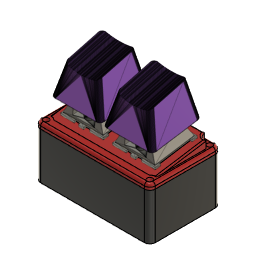
BFDeck x2 v6 (Autodesk Fusion 360 design; units mm, degrees)
Autodesk Fusion 360 part; units mm, degrees
sketch "Sketch1" plane through (0, 0, 0) normal (0, 0, 1) x (1, 0, 0)
  line L0 (2, 0) -> (40, 0)
  line L1 (42, 2) -> (42, 24)
  line L2 (40, 26) -> (2, 26)
  line L3 (0, 24) -> (0, 2)
  arc A0 (2, 26) -> (0, 24) centre (2, 24) ccw
  arc A1 (42, 24) -> (40, 26) centre (40, 24) ccw
  arc A2 (40, 0) -> (42, 2) centre (40, 2) ccw
  arc A3 (0, 2) -> (2, 0) centre (2, 2) ccw
  point P0 (42, 0)
  point P1 (42, 26)
  dimension "d1" = 42
  dimension "d2" = 26
  dimension "d3" = 2
  dimension "d4" = 2
  dimension "d5" = 2
  dimension "d6" = 2
  constraint horizontal L0
  constraint vertical L1
  constraint horizontal L2
  constraint vertical L3
  constraint tangent L2 A0
  constraint tangent L3 A0
  constraint coincident P1 L1
  constraint coincident P1 L2
  constraint tangent L1 A1
  constraint tangent L2 A1
  constraint coincident P0 L0
  constraint coincident P0 L1
  constraint tangent L0 A2
  constraint tangent L1 A2
  constraint coincident origin L0
  constraint coincident origin L3
  constraint tangent L0 A3
  constraint tangent L3 A3
  measures "d1" distance of origin P0
  measures "d2" distance of P0 P1
  measures "d3" radius of A0
  measures "d4" radius of A1
  measures "d5" radius of A2
  measures "d6" radius of A3
extrude "Extrude1" add sketch "Sketch1" along normal blind 2 makes body 1
sketch "Sketch2" plane through (0, 0, 2) normal (0, 0, 1) x (-1, 0, 0)
  arc A0 (0, -2) -> (-2, 0) centre (-2, -2) ccw
  line L0 (-2, 0) -> (-40, 0)
  arc A1 (-40, 0) -> (-42, -2) centre (-40, -2) ccw
  line L1 (-42, -2) -> (-42, -24)
  arc A2 (-42, -24) -> (-40, -26) centre (-40, -24) ccw
  line L2 (-40, -26) -> (-2, -26)
  arc A3 (-2, -26) -> (0, -24) centre (-2, -24) ccw
  line L3 (0, -24) -> (0, -2)
  line L4 (-21, -26) -> (-21, 0)
  line L5 (0, -13) -> (-42, -13)
  line L6 (-40, -24) -> (-2, -24)
  line L7 (-2, -24) -> (-2, -2)
  line L8 (-2, -2) -> (-40, -2)
  line L9 (-40, -2) -> (-40, -24)
  line L10 (-40, -24) -> (-2, -2) construction
  line L11 (-2, -24) -> (-40, -2) construction
  circle A4 centre (-2, -24) radius 2
  circle A5 centre (-40, -24) radius 2
  circle A6 centre (-40, -2) radius 2
  circle A7 centre (-2, -2) radius 2
  circle A8 centre (-2, -24) radius 1
  circle A9 centre (-40, -24) radius 1
  circle A10 centre (-40, -2) radius 1
  circle A11 centre (-2, -2) radius 1
  point P0 (-21, -13)
  constraint midpoint L2 L4.start
  constraint midpoint L0 L4.end
  constraint midpoint L3 L5.start
  constraint midpoint L1 L5.end
  constraint horizontal L6
  constraint perpendicular L6 L7
  constraint parallel L6 L8
  constraint parallel L7 L9
  constraint coincident A2.centre L6.start
  constraint coincident L10 P0
  constraint coincident L11 P0
  constraint midpoint L4 P0
  constraint concentric A3 A4
  constraint concentric A1 A6
  constraint concentric A0 A7
  constraint concentric A4 A8
  constraint concentric A5 A9
  constraint concentric A6 A10
  constraint concentric A7 A11
extrude "Extrude2" add sketch "Sketch2" along normal blind 15 contours A0 L7 L8 A7 A11 | L3 L5 L7 A7 | L0 L4 L8 A7 | L3 L5 L7 A4 | L7 L8 A7 A11 | L0 L4 L8 A6 | A3 L6 L7 A4 A8 | A1 L8 L9 A6 A10 | L2 L4 L6 A4 | L6 L7 A4 A8 | L1 L5 L9 A6 | L8 L9 A6 A10 | L2 L4 L6 A5 | L1 L5 L9 A5 | A2 L6 L9 A5 A9 | L6 L9 A5 A9 bodies 1
sketch "Sketch1 (2)" plane through (0, 0, 17) normal (0, 0, 1) x (-1, 0, 0) in component "Component"
  circle A0 centre (-40, -2) radius 1
  circle A1 centre (-2, -2) radius 1
  circle A2 centre (-40, -24) radius 1
  line L0 (-4, -24) -> (-38, -24)
  arc A3 (-38, -24) -> (-40, -22) centre (-40, -24) ccw
  line L1 (-40, -22) -> (-40, -4)
  arc A4 (-40, -4) -> (-38, -2) centre (-40, -2) ccw
  line L2 (-38, -2) -> (-4, -2)
  arc A5 (-4, -2) -> (-2, -4) centre (-2, -2) ccw
  line L3 (-2, -4) -> (-2, -22)
  arc A6 (-2, -22) -> (-4, -24) centre (-2, -24) ccw
  circle A7 centre (-2, -24) radius 1
  arc A8 (0, -2) -> (-2, 0) centre (-2, -2) ccw
  line L4 (-2, 0) -> (-40, 0)
  arc A9 (-40, 0) -> (-42, -2) centre (-40, -2) ccw
  line L5 (-42, -2) -> (-42, -24)
  arc A10 (-42, -24) -> (-40, -26) centre (-40, -24) ccw
  line L6 (-40, -26) -> (-2, -26)
  arc A11 (-2, -26) -> (0, -24) centre (-2, -24) ccw
  line L7 (0, -24) -> (0, -2)
  line L8 (0, -22) -> (-34, -22)
  line L9 (-34, -22) -> (-34, 0)
  line L10 (-34, 0) -> (0, 0)
  line L11 (0, 0) -> (0, -22)
  circle A12 centre (-2, -24) radius 2
  circle A13 centre (-40, -24) radius 2
  circle A14 centre (-40, -2) radius 2
  circle A15 centre (-2, -2) radius 2
  circle A16 centre (-2, -24) radius 1
  circle A17 centre (-40, -24) radius 1
  circle A18 centre (-40, -2) radius 1
  circle A19 centre (-2, -2) radius 1
  dimension "d31" = 34
  constraint horizontal L8
  constraint vertical L9
  constraint horizontal L10
  constraint vertical L11
  constraint concentric A6 A12
  constraint coincident L6.end A12
  constraint concentric A2 A13
  constraint coincident A10.end A13
  constraint concentric A0 A14
  constraint coincident A9.end A14
  constraint concentric A1 A15
  constraint coincident A8.start A15
  constraint tangent L11 A15
  constraint concentric A12 A16
  constraint concentric A13 A17
  constraint concentric A14 A18
  constraint concentric A15 A19
  measures "d31" distance of L9.end L10.end
extrude "Extrude1'" add sketch "Sketch1 (2)" along normal blind 2 separate body contours L0 L6 A12 A13 | L0 A3 L1 A4 L2 A6 L8 L9 A12 A13 A14 | A6 A11 A12 | A3 A10 A13 | L2 A5 L3 L8 L9 A15 | L3 L7 L8 L11 A15 | L7 L8 A12 | L1 L5 A13 A14 | A5 A8 A15 | A4 A9 A14 | L2 L4 L9 L10 A15 | L2 L4 L9 A14 makes body 2 in component "Component"
fillet "Fillet1" radius 1 8 edges at (21, 26, 19) (0.5858, 25.4142, 19) (0, 23, 19) (0.5858, 0.5858, 19) (21, 0, 19) (41.4142, 0.5858, 19) (42, 13, 19) (41.4142, 25.4142, 19) on bodies 2 in component "Component"
ref_plane "WorkPlane1" through (1.5, 0, 0) normal (1, 0, 0) x (0, 1, 0) in component "Component"
sketch "Sketch2 (2)" plane through (1.5, 0, 0) normal (1, 0, 0) x (0, 1, 0) in component "Component"
  line L0 (0, 18.7929) -> (26, 18.7929)
  line L1 (2, 18.7929) -> (24, 22.238)
  line L2 (24, 19) -> (2, 19)
  line L3 (24, 22.238) -> (24, 19)
  point P0 (1, 19)
  dimension "d17" = 2
  dimension "d18" = 26
  dimension "d19" = 2
  dimension "d20" = 8.9
  constraint horizontal L0
  constraint coincident L0 L1.start
  constraint coincident L2.start L3.end
  constraint perpendicular L0 L3
  measures "d17" horizontal distance of L0.end L1.end
  measures "d18" distance of L0.start L0.end
  measures "d19" distance of L0.start L1.start
  measures "d20" angle of L1 L2
extrude "Extrude2'" add sketch "Sketch2 (2)" along normal blind 39 bodies 2 in component "Component"
sketch "Sketch3" plane through (0, 0, 19) normal (0, 0, 1) x (-1, 0, 0) in component "Component"
  arc A0 (-1, -24) -> (-1.5, -23.134) centre (-2, -24) ccw
  arc A1 (-2, -1) -> (-1, -2) centre (-2, -2) ccw
  circle A2 centre (-2, -24) radius 2
  circle A3 centre (-40, -24) radius 2
  circle A4 centre (-2, -2) radius 2
  circle A5 centre (-40, -2) radius 2
  line L0 (-1.5, -3.3227) -> (-1.5, -23.134)
  line L1 (-1, -24) -> (-1, -22)
  line L2 (-40.5, -23.134) -> (-40.5, -3.3227)
  line L3 (-40.5, -3.3227) -> (-1.5, -3.3227)
  line L4 (-1, -22) -> (-1, -2)
  line L5 (-2, -1) -> (-40, -1)
  arc A6 (-41, -2) -> (-40, -1) centre (-40, -2) ccw
  line L6 (-41, -2) -> (-41, -24)
  arc A7 (-40.5, -23.134) -> (-41, -24) centre (-40, -24) ccw
  dimension "d23" = 4
  dimension "d24" = 4
  dimension "d25" = 4
  dimension "d26" = 4
  constraint concentric A0 A2
  constraint concentric A1 A4
  constraint coincident A3.centre A7.centre
  constraint coincident A5.centre A6.centre
  measures "d23" diameter of A2
  measures "d24" diameter of A3
  measures "d25" diameter of A4
  measures "d26" diameter of A5
extrude "Extrude3" cut sketch "Sketch3" along normal blind 4 contours A0 A2 L0 L1 | A0 A2 L0 L1 | A1 A4 L0 L3 L4 L5 | A4 L0 L3 | A1 A4 L4 L5 | A5 L2 L3 L5 A6 L6 | A5 L2 L3 | A5 L5 A6 L6 | A3 L2 L6 A7 | A3 L2 L6 A7 bodies 2 in component "Component"
fillet "Fillet2" radius 0.5 5 edges at (1.5, 13, 20.5154) (21, 24, 22.238) (40.5, 13, 20.5154) (38.7753, 22.4189, 21.9904) (3.2247, 22.4189, 21.9904) on bodies 2 in component "Component"
sketch "Sketch4" plane through (0, -2.8246, 18.0374) normal (0, -0.15471, 0.98796) x (1, 0, 0) in component "Component"
  line L0 (3.5002, 6.2221) -> (38.4998, 6.2221)
  line L1 (21, 26.5671) -> (21, 6.2221)
  line L2 (21, 16.3946) -> (36.5265, 16.3946)
  line L3 (21, 16.3946) -> (2, 16.3946)
  line L4 (40, 6.9077) -> (40, 24.5427)
  line L5 (37.5505, 26.5671) -> (4.4495, 26.5671)
  ellipse E0 centre (2, 27.0732) end of major axis (2, 24.5427) minor radius 2.5 (2, 24.5427) -> (4.4495, 26.5671) ccw
  line L6 (2, 24.5427) -> (2, 6.9077)
  line L7 (18.5, 23.3946) -> (4.5, 23.3946)
  line L8 (4.5, 23.3946) -> (4.5, 9.3946)
  line L9 (4.5, 9.3946) -> (18.5, 9.3946)
  line L10 (18.5, 9.3946) -> (18.5, 23.3946)
  line L11 (18.5, 23.3946) -> (4.5, 9.3946) construction
  line L12 (4.5, 23.3946) -> (18.5, 9.3946) construction
  line L13 (23.5, 9.3946) -> (23.5, 23.3946)
  line L14 (23.5, 23.3946) -> (37.5, 23.3946)
  line L15 (37.5, 23.3946) -> (37.5, 9.3946)
  line L16 (37.5, 9.3946) -> (23.5, 9.3946)
  ellipse E1 centre (2, 4.8834) end of major axis (2, 2.859) minor radius 2 (3.5002, 6.2221) -> (2, 6.9077) ccw
  ellipse E2 centre (40, 27.0732) end of major axis (40, 24.5427) minor radius 2.5 (37.5505, 26.5671) -> (40, 24.5427) ccw
  ellipse E3 centre (40, 4.8834) end of major axis (40, 2.859) minor radius 2 (40, 6.9077) -> (38.4998, 6.2221) ccw
  point P0 (11.5, 16.3946)
  dimension "d32" = 14
  dimension "d33" = 20.345
  dimension "d45" = 5
  constraint midpoint L0 L1.end
  constraint midpoint L1 L2.start
  constraint horizontal L7
  constraint perpendicular L7 L8
  constraint parallel L7 L9
  constraint parallel L8 L10
  constraint coincident L11 P0
  constraint coincident L12 P0
  constraint midpoint L3 P0
  constraint equal L9 L10
  constraint parallel L0 L3
  constraint parallel L1 L10
  constraint symmetric L1 L7.start L13.end
  constraint symmetric L1 L7.end L14.end
  constraint symmetric L1 L8.end L15.end
  constraint symmetric L1 L9.end L13.start
  constraint parallel L2 L3
  measures "d32" distance of L8.end L9.end
  measures "d33" vertical distance of L1.start L1.end
  measures "d45" distance of L10 L13
extrude "Extrude4" cut sketch "Sketch4" against normal blind 5 contours L3 L8 L9 L10 | L3 L7 L8 L10 | L13 L14 L15 L16 bodies 2 in component "Component"
ref_plane "WorkPlane1" through (21, 13.8934, 19.1371) normal (0, -0.15471, 0.98796) x (0, -0.98796, -0.15471)
sketch "Sketch3 (2)" plane through (17, 10.975, 18.6801) normal (0, -0.15471, 0.98796) x (0, -0.98796, -0.15471)
  line L0 (-10.6617, -13) -> (5.3383, -13)
  line L1 (5.3383, -13) -> (5.3383, 18.5)
  line L2 (5.3383, 18.5) -> (-10.6617, 18.5)
  line L3 (-10.6617, 18.5) -> (-10.6617, -13)
  line L4 (-9.6617, 20.5) -> (-9.6617, 6.5)
  line L5 (-9.6617, 20.5) -> (4.3383, 20.5)
  line L6 (-9.6617, -12.5) -> (4.3383, -12.5)
  dimension "d42" = 31.5
  dimension "d43" = 1
  dimension "d44" = 16
  dimension "d47" = 0.5
  constraint horizontal L0
  constraint vertical L1
  constraint horizontal L2
  constraint vertical L3
  measures "d42" distance of L0.start L2.end
  measures "d43" distance of L3 L4
  measures "d44" distance of L1.end L2.end
  measures "d47" distance of L0 L6
extrude "Extrude5" cut sketch "Sketch3 (2)" against normal blind 4 bodies 2 in component "Component"
other "Base Mesh Feature2"
other "Modify5"
other "Modify6"
other "Modify7"
other "Modify8"
other "Modify9"
other "CopyPasteMeshes2"
other "Modify10"
other "Modify11"
other "Modify12"
other "Base Mesh Feature3"
other "Modify13"
other "Modify14"
other "Modify15"
other "Modify16"
other "Modify17"
other "Modify18"
other "Modify19"
other "CopyPasteMeshes3"
other "Modify20"
sketch "Sketch4 (2)" plane through (0, 26, 0) normal (0, 1, 0) x (-1, 0, 0)
  line L0 (-40, 0) -> (-2, 0)
  line L1 (-2, 0) -> (-2, 17)
  line L2 (-2, 17) -> (-40, 17)
  line L3 (-40, 17) -> (-40, 0)
  line L4 (-25.25, 6) -> (-16.75, 6)
  line L5 (-16.75, 6) -> (-16.75, 3)
  line L6 (-16.75, 3) -> (-25.25, 3)
  line L7 (-25.25, 3) -> (-25.25, 6)
  line L8 (-21, 0) -> (-21, 12)
  dimension "d49" = 8.5
  dimension "d50" = 3
  dimension "d51" = 3
  constraint horizontal L4
  constraint vertical L5
  constraint horizontal L6
  constraint vertical L7
  constraint midpoint L0 L8.start
  constraint perpendicular L0 L8
  constraint midpoint L4 L8
  measures "d49" distance of L4.start L4.end
  measures "d50" distance of L4.end L5.end
  measures "d51" distance of L0 L6
extrude "Extrude3'" cut sketch "Sketch4 (2)" against normal blind 4 contours L4 L6 L7 L8 | L4 L5 L6 L8 bodies 1
sketch "Sketch5" plane through (0, 24, 0) normal (0, -1, 0) x (1, 0, 0)
  line L0 (16.75, 3) -> (16.75, 6)
  line L1 (16.75, 6) -> (25.25, 6)
  line L2 (25.25, 6) -> (25.25, 3)
  line L3 (25.25, 3) -> (16.75, 3)
  line L4 (4, 2) -> (38, 2)
  line L5 (38, 2) -> (38, 17)
  line L6 (38, 17) -> (4, 17)
  line L7 (4, 17) -> (4, 2)
  line L8 (12, 6) -> (30, 6)
  line L9 (30, 6) -> (30, 2)
  line L10 (30, 2) -> (12, 2)
  line L11 (12, 2) -> (12, 6)
  dimension "d55" = 18
  constraint horizontal L8
  constraint vertical L9
  constraint horizontal L10
  constraint vertical L11
  constraint midpoint L1 L8
  constraint collinear L4 L10
  measures "d55" distance of L8.start L8.end
extrude "Extrude4'" cut sketch "Sketch5" against normal blind 1 contours L0 L2 L3 L4 L8 L9 L10 L11 bodies 1
component "Component" placed x (1, 0, 0) y (0, 1, 0) z (0, 0, 1) at (0, 0, 0)
